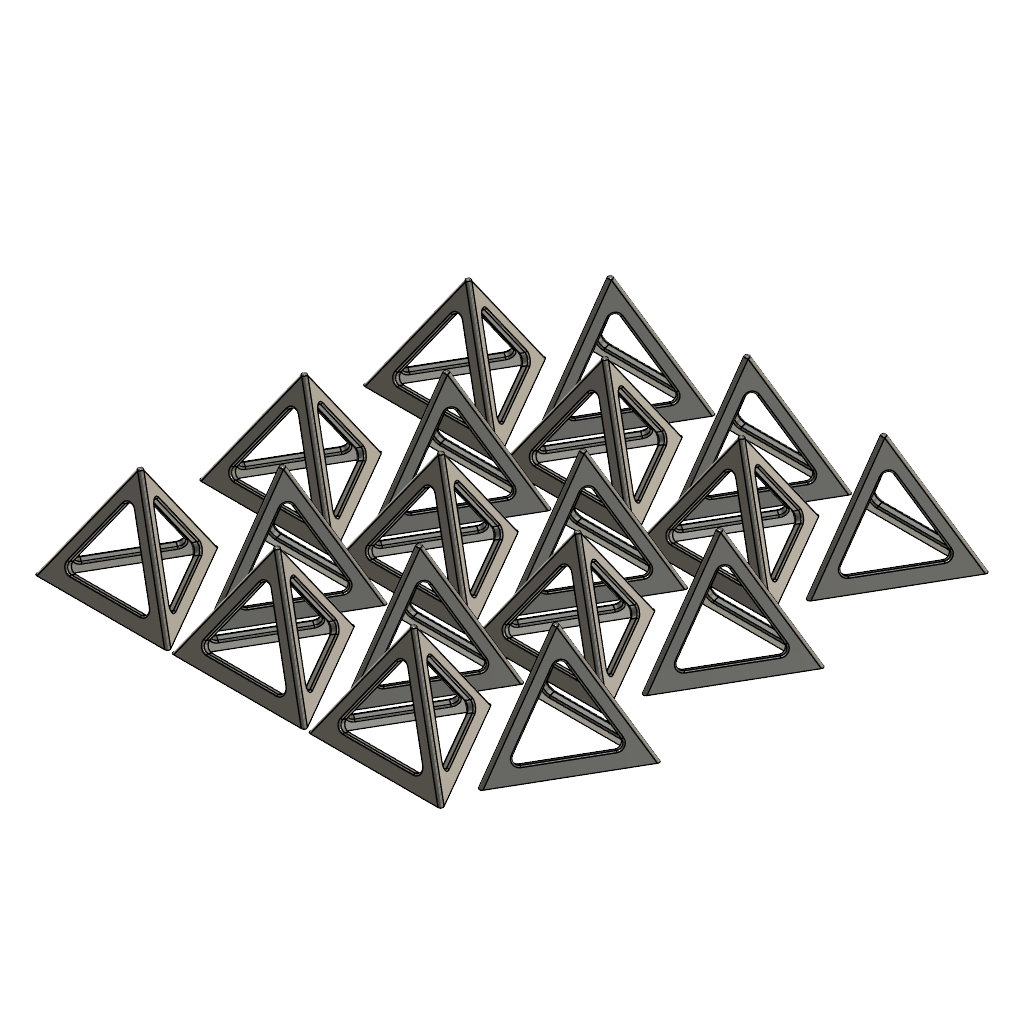
3D printable painters tripod (Autodesk Fusion 360 design; units mm, degrees)
part number: 2026-09-18-09-55-47-208
part number: 2026-09-18-09-56-40-934
Autodesk Fusion 360 part; units mm, degrees
note: some values were not read from the file. Chosen so that the rebuilt part matches the saved one: which bodies a step acts on; which face or edge a step refers to.
sketch "Base profile" plane through (0, 0, 0) normal (0, 0, 1) x (1, 0, 0) in component "Painters tripod"
  line L0 (-25, -14.4338) -> (0, 28.8675)
  line L1 (0, 28.8675) -> (25, -14.4338)
  line L2 (25, -14.4338) -> (-25, -14.4338)
  line L3 (12.5, 7.2169) -> (-25, -14.4338) construction
  line L4 (0, -14.4338) -> (0, 28.8675) construction
  dimension "d1" = 50
  constraint horizontal L2
  constraint equal L0 L1
  constraint equal L1 L2
  constraint midpoint L1 L3.start
  constraint midpoint L2 L4.start
  constraint coincident L3 origin
  constraint coincident L4 origin
  measures "d1" distance of L0.start L0.end
ref_plane "WorkPlane1" through (0, 0, 40.8248) normal (0, 0, 1) x (1, 0, 0) in component "Painters tripod"
sketch "loft profile" plane through (0, 0, 40.8248) normal (0, 0, 1) x (1, 0, 0) in component "Painters tripod"
loft "Loft1" add profiles "Base profile" section 1 section 2 point at (0, 0, 40.8248) makes body 1 in component "Painters tripod"
shell "Shell1" thickness 2.5 removed faces 1 at (0, 0, 0) on bodies 1 in component "Painters tripod"
sketch "Sketch3" plane through (0, -12.83, 4.5361) normal (0, -0.942809, 0.333333) x (1, 0, 0) in component "Painters tripod"
  line L0 (-25, -4.8113) -> (25, -4.8113)
  line L1 (25, -4.8113) -> (0, 38.49)
  line L2 (0, 38.49) -> (-25, -4.8113)
  line L3 (-16.3397, 0.1887) -> (16.3397, 0.1887)
  line L4 (16.3397, 0.1887) -> (0, 28.49)
  line L5 (0, 28.49) -> (-16.3397, 0.1887)
  dimension "d5" = -5
extrude "Extrude1" cut sketch "Sketch3" against normal up to surface (2.5 mm away) contours L3 L4 L5 bodies 1 in component "Painters tripod"
pattern_circular "C-Pattern1" count 3 over 360 about axis through (0, 0, 1.75) along (0, 0, 1) of "Extrude1" in component "Painters tripod"
fillet "Fillet1" radius 1 3 edges at (0, 14.4338, 20.4124) (12.5, -7.2169, 20.4124) (-12.5, -7.2169, 20.4124) on bodies 1 in component "Painters tripod"
fillet "Fillet1" radius 0.5 18 edges at (0, -12.7671, 4.714) (0, -10.4101, 3.8807) (11.0566, 6.3835, 4.714) (9.0154, 5.205, 3.8807) (-9.0154, 5.205, 3.8807) (-11.0566, 6.3835, 4.714) (-11.0566, -3.0502, 18.0554) (-9.0154, -4.2287, 17.2221) (-2.8868, 11.1004, 18.0554) (-0.8455, 9.9219, 17.2221) (0.8455, 9.9219, 17.2221) (2.8868, 11.1004, 18.0554) (9.0154, -4.2287, 17.2221) (11.0566, -3.0502, 18.0554) (8.1699, -5.6932, 17.2221) (8.1699, -8.0502, 18.0554) (-8.1699, -8.0502, 18.0554) (-8.1699, -5.6932, 17.2221) on bodies 1 in component "Painters tripod"
fillet "Fillet1" radius 2 9 edges at (1.8661, 19.9449, 4.2974) (-1.8661, 19.9449, 4.2974) (1.8661, 1.0774, 30.9801) (-1.8661, 1.0774, 30.9801) (0, -2.1548, 30.9801) (-18.2059, -8.3563, 4.2974) (-16.3397, -11.5886, 4.2974) (16.3397, -11.5886, 4.2974) (18.2059, -8.3563, 4.2974) on bodies 1 in component "Painters tripod"
pattern_linear "R-Pattern1" count 6 spacing 50 along (1, 0, 0) of bodies 1 makes body 2 at (64.2129, 3.25, 1.4142) makes body 3 at (114.2129, 3.25, 1.4142) makes body 4 at (164.2129, 3.25, 1.4142) makes body 5 at (214.2129, 3.25, 1.4142) makes body 6 at (264.2129, 3.25, 1.4142) in component "Painters tripod"
move_body "Move14" bodies 6 to x (0.5, -0.866025, 0) y (0.866025, 0.5, 0) z (0, 0, 1) at (125.3323, 188.2143, 0) in component "Painters tripod"
move_body "Move15" bodies 6 to x (1, 0, 0) y (0, 1, 0) z (0, 0, 1) at (-225, 55, 0) in component "Painters tripod"
move_body "Move16" bodies 5 to x (0.5, -0.866025, 0) y (0.866025, 0.5, 0) z (0, 0, 1) at (100.3323, 144.9131, 0) in component "Painters tripod"
move_body "Move17" bodies 5 to x (1, 0, 0) y (0, 1, 0) z (0, 0, 1) at (-125, 55, 0) in component "Painters tripod"
move_body "Move18" bodies 4 to x (0.5, -0.866025, 0) y (0.866025, 0.5, 0) z (0, 0, 1) at (75.3323, 101.6118, 0) in component "Painters tripod"
move_body "Move19" bodies 4 to x (1, 0, 0) y (0, 1, 0) z (0, 0, 1) at (-25, 55, 0) in component "Painters tripod"
pattern_linear "R-Pattern3" count 3 spacing 60 along (0, 1, 0) of bodies 1 6 2 5 3 4 makes body 7 at (14.2129, 63.25, 1.4142) makes body 8 at (-4.2919, 106.0662, 1.4142) makes body 9 at (64.2129, 63.25, 1.4142) makes body 10 at (45.7081, 106.0662, 1.4142) makes body 11 at (114.2129, 63.25, 1.4142) makes body 12 at (114.2129, 123.25, 1.4142) makes body 13 at (111.1193, 83.458, 1.4142) makes body 14 at (139.5452, 143.458, 1.4142) makes body 15 at (89.5452, 83.458, 1.4142) makes body 16 at (85.2533, 136.0242, 1.4142) makes body 17 at (11.1193, 83.458, 1.4142) makes body 18 at (11.1193, 143.458, 1.4142) in component "Painters tripod"
component "Painters tripod" placed x (1, 0, 0) y (0, 1, 0) z (0, 0, 1) at (0, 0, 0)
equation "d2 = ( d1 * sqrt(6) ) / 3"
equation "d18 = d1"
